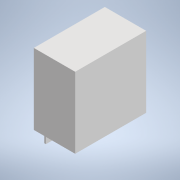
# Autodesk Inventor part: camera
Saved by Autodesk Inventor 2022 (Build 260153000, 153)
## iProperties
Created: 2024-10-13
Part Number: camera
Material: Типовые
Document SubType Name: Modeling
Designer: Andrey
Density: 1 g/cm^3
Appearance: По умолчанию
Author: Andrey
Autodesk Inventor part; units mm, degrees
ref_plane "YZ Plane" through (0, 0, 0) normal (1, 0, 0) x (0, 1, 0)
ref_plane "XZ Plane" through (0, 0, 0) normal (0, 1, 0) x (-1, 0, 0)
ref_plane "XY Plane" through (0, 0, 0) normal (0, 0, 1) x (1, 0, 0)
sketch "Эскиз1" plane through (0, 0, 0) normal (1, 0, 0) x (0, 1, 0)
  line L0 (-4.25, 4.25) -> (4.25, 4.25)
  line L1 (4.25, 4.25) -> (4.25, -4.25)
  line L2 (4.25, -4.25) -> (-4.25, -4.25)
  line L3 (-4.25, -4.25) -> (-4.25, 4.25)
  line L4 (-4.25, 4.25) -> (4.25, -4.25) construction
  line L5 (4.25, 4.25) -> (-4.25, -4.25) construction
  point P0 (0, 0)
  dimension "d0" = 8.5
  dimension "d1" = 8.5
  constraints: 12 end point, 2 midpoint, 2 parallel, 1 horizontal, 1 perpendicular
  measures "d0" distance of L1.end L2.end
  measures "d1" distance of L0.end L1.end
extrude "Выдавливание1" add sketch "Эскиз1" along normal blind 4.95
sketch "Эскиз2" plane through (0, -4.25, -4.25) normal (0, -1, 0) x (1, 0, 0)
  line L0 (0.2, 7.25) -> (0, 7.25)
  line L1 (0, 7.25) -> (0, 1.25)
  line L2 (0, 1.25) -> (0.2, 1.25)
  line L3 (0.2, 1.25) -> (0.2, 7.25)
  line L4 (0.2, 7.25) -> (0, 1.25) construction
  line L5 (0, 7.25) -> (0.2, 1.25) construction
  line L6 (0, 8.5) -> (0, 0) projected
  point P0 (0, 4.25)
  point P1 (0.1, 4.25)
  point P2 (0, 4.25)
  dimension "d4" = 0.2
  dimension "d5" = 6
  constraints: 12 end point, 4 midpoint, 2 parallel, 1 horizontal, 1 perpendicular
  measures "d4" distance of L2.end L1.end
  measures "d5" distance of L1.end L0.end
extrude "Выдавливание2" add sketch "Эскиз2" along normal blind 2
